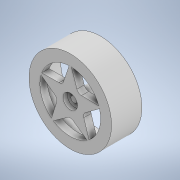
# Autodesk Inventor part: Колесо красивое
Saved by Autodesk Inventor 2022 (Build 260153000, 153)
## iProperties
Created: 2022-07-10
Part Number: Колесо красивое
Material: Типовые
Document SubType Name: Modeling
Designer: Константин
Density: 1 g/cm^3
Appearance: По умолчанию
Author: Константин
Autodesk Inventor part; units mm, degrees
ref_plane "YZ Plane" through (0, 0, 0) normal (1, 0, 0) x (0, 1, 0)
ref_plane "XZ Plane" through (0, 0, 0) normal (0, 1, 0) x (-1, 0, 0)
ref_plane "XY Plane" through (0, 0, 0) normal (0, 0, 1) x (1, 0, 0)
sketch "Эскиз1" plane through (0, 0, 0) normal (0, 0, 1) x (1, 0, 0)
  circle A0 centre (0, 0) radius 34
  circle A1 centre (0, 0) radius 33
  dimension "d0" = 68
  dimension "d1" = 66
  constraints: 2 centre point, 2 coincident
  measures "d0" diameter of A0
  measures "d1" diameter of A1
extrude "Выдавливание1" add sketch "Эскиз1" along normal blind 25
sketch "Эскиз4" plane through (0, 0, 25) normal (0, 0, 1) x (1, 0, 0)
  circle A0 centre (0, 0) radius 33
  constraints: 1 centre point, 1 coincident
extrude "Выдавливание2" add sketch "Эскиз4" against normal blind 6
sketch "Эскиз5" plane through (0, 0, 25) normal (0, 0, 1) x (1, 0, 0)
  circle A0 centre (0, 0) radius 25
  line L0 (0, 25) -> (23.7764, 7.7254)
  line L1 (23.7764, 7.7254) -> (14.6946, -20.2254)
  line L2 (14.6946, -20.2254) -> (-14.6946, -20.2254)
  line L3 (-14.6946, -20.2254) -> (-23.7764, 7.7254)
  line L4 (-23.7764, 7.7254) -> (0, 25)
  circle A1 centre (0, 0) radius 11
  line L5 (0, 25) -> (-4.9275, 9.8346)
  line L6 (0, 25) -> (4.9275, 9.8346)
  line L7 (23.7764, 7.7254) -> (7.8306, 7.7254)
  line L8 (23.7764, 7.7254) -> (10.876, -1.6473)
  line L9 (14.6946, -20.2254) -> (9.7671, -5.06)
  line L10 (14.6946, -20.2254) -> (1.7942, -10.8527)
  line L11 (-14.6946, -20.2254) -> (-1.7942, -10.8527)
  line L12 (-14.6946, -20.2254) -> (-9.7671, -5.06)
  line L13 (-7.8306, 7.7254) -> (-23.7764, 7.7254)
  line L14 (-10.876, -1.6473) -> (-23.7764, 7.7254)
  line L15 (4.9275, 9.8346) -> (9.7671, -5.06)
  line L16 (10.876, -1.6473) -> (-1.7942, -10.8527)
  line L17 (1.7942, -10.8527) -> (-10.876, -1.6473)
  line L18 (-9.7671, -5.06) -> (-4.9275, 9.8346)
  line L19 (-7.8306, 7.7254) -> (7.8306, 7.7254)
  line L20 (-7.8306, 7.7254) -> (-4.9275, 9.8346)
  line L21 (-6.3791, 8.78) -> (0, 27.7353)
  line L22 (4.9275, 9.8346) -> (7.8306, 7.7254)
  line L23 (10.876, -1.6473) -> (9.7671, -5.06)
  line L24 (1.7942, -10.8527) -> (-1.7942, -10.8527)
  line L25 (-9.7671, -5.06) -> (-10.876, -1.6473)
  line L26 (0, 27.7353) -> (6.3791, 8.78)
  line L27 (-10.3215, -3.3537) -> (-26.3778, 8.5707)
  line L28 (-26.3778, 8.5707) -> (-6.3791, 8.78)
  line L29 (0, -10.8527) -> (-16.3024, -22.4383)
  line L30 (-16.3024, -22.4383) -> (-10.3215, -3.3537)
  line L31 (10.3215, -3.3537) -> (16.3024, -22.4383)
  line L32 (16.3024, -22.4383) -> (0, -10.8527)
  line L33 (6.3791, 8.78) -> (26.3778, 8.5707)
  line L34 (26.3778, 8.5707) -> (10.3215, -3.3537)
  point P0 (23.7764, 7.7254)
  point P1 (23.7764, 7.7254)
  point P2 (-15.4339, -19.6671)
  point P3 (-10.3966, -3.5932)
  point P4 (-10.523, -3.204)
  point P5 (-24.0463, 6.8392)
  point P6 (0.2046, -10.9981)
  point P7 (-0.2046, -10.9981)
  point P8 (-13.9352, -20.756)
  point P9 (13.9352, -20.756)
  point P10 (10.523, -3.204)
  point P11 (10.3966, -3.5932)
  point P12 (15.4339, -19.6671)
  point P13 (24.0463, 6.8392)
  point P14 (23.4738, 8.6011)
  point P15 (0.9263, 24.9828)
  point P16 (6.299, 9.0179)
  point P17 (6.63, 8.7774)
  point P18 (-23.4738, 8.6011)
  point P19 (-6.63, 8.7774)
  point P20 (-6.299, 9.0179)
  point P21 (-0.9263, 24.9828)
  dimension "d8" = 22
  dimension "d7" = 50
  dimension "d15" = 360
  constraints: 70 end point, 3 coincident, 3 horizontal, 2 midpoint, 2 point on circle, 1 centre point, 1 collinear, 50 other
  measures "d7" diameter of A0
extrude "Выдавливание3" cut sketch "Эскиз5" against normal through all contours A0 L31 L1 L34 | L1 L31 A1 L34 | L33 L0 L26 A0 | L33 A1 L26 L0 | A0 L29 L2 L32 | L2 L29 A1 L32 | L21 L4 L28 A0 | L21 A1 L28 L4 | A0 L27 L3 L30 | L3 L27 A1 L30
fillet "Сопряжение1" radius 4 10 edges at (6.299, 9.0179, 22) (6.63, 8.7774, 22) (10.523, -3.204, 22) (10.3966, -3.5932, 22) (0.2046, -10.9981, 22) (-0.2046, -10.9981, 22) (-10.523, -3.204, 22) (-10.3966, -3.5932, 22) (-6.299, 9.0179, 22) (-6.63, 8.7774, 22)
sketch "Эскиз6" plane through (0, 0, 25) normal (0, 0, 1) x (1, 0, 0)
  circle A0 centre (0, 0) radius 6
  dimension "d18" = 12
  constraints: 1 centre point, 1 coincident
  measures "d18" diameter of A0
extrude "Выдавливание4" cut sketch "Эскиз6" against normal blind 5.5
sketch "Эскиз7" plane through (0, 0, 19.5) normal (0, 0, 1) x (1, 0, 0)
  circle A0 centre (0, 0) radius 2.5
  dimension "d21" = 5
  constraints: 1 centre point, 1 coincident
  measures "d21" diameter of A0
extrude "Выдавливание5" add sketch "Эскиз7" along normal blind 2.5
fillet "Сопряжение2" radius 2 1 edges at (-6, 0, 19.5)
sketch "Эскиз8" plane through (0, 0, 19) normal (0, 0, -1) x (-1, 0, 0)
  circle A0 centre (0, 0) radius 4 projected
  circle A1 centre (0, 0) radius 4.5
  dimension "d25" = 9
  constraints: 1 centre point, 1 coincident
  measures "d25" diameter of A1
extrude "Выдавливание6" add sketch "Эскиз8" along normal blind 23 contours A0
sketch "Эскиз9" plane through (0, 0, -4) normal (0, 0, -1) x (-1, 0, 0)
  circle A0 centre (0, 0) radius 2.5
  dimension "d28" = 5
  constraints: 1 centre point, 1 coincident
  measures "d28" diameter of A0
extrude "Выдавливание7" add sketch "Эскиз9" along normal blind 3.5
sketch "Эскиз10" plane through (0, 0, -7.5) normal (0, 0, -1) x (-1, 0, 0)
  circle A0 centre (0, 0) radius 1
  dimension "d31" = 2
  constraints: 1 centre point, 1 coincident
  measures "d31" diameter of A0
extrude "Выдавливание8" cut sketch "Эскиз10" against normal blind 10
